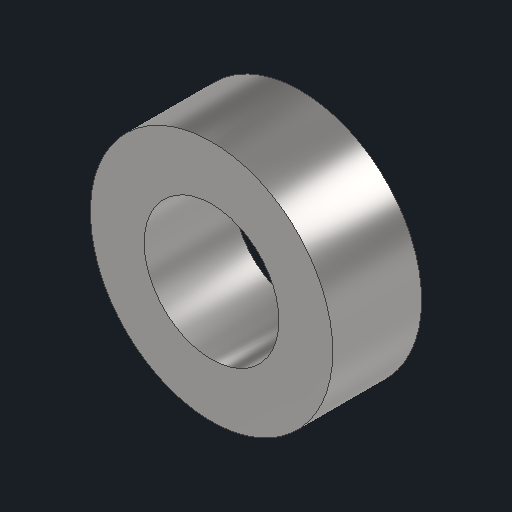
# Autodesk Inventor part: small_bearing
Saved by Autodesk Inventor 2023 (Build 270158000, 158)
## iProperties
Created: 2024-04-13
Part Number: small_bearing
Material: Steel, Alloy
Document SubType Name: Modeling
Designer: szymo
Density: 7.73 g/cm^3
Appearance: Semi-Polished
Mass: 1.12194 g
Surface Area: 2.33106 cm^2
Volume: 0.145142 cm^3
Author: szymo
Autodesk Inventor part; units mm, degrees
ref_plane "YZ Plane" through (0, 0, 0) normal (1, 0, 0) x (0, 1, 0)
ref_plane "XZ Plane" through (0, 0, 0) normal (0, 1, 0) x (-1, 0, 0)
ref_plane "XY Plane" through (0, 0, 0) normal (0, 0, 1) x (1, 0, 0)
sketch "Sketch1" plane through (0, 0, 0) normal (0, 0, 1) x (1, 0, 0)
  circle A0 centre (2.5, 0) radius 2.5 projected
  circle A1 centre (2.5, 0) radius 4.5
  point P0 (0, 0)
  dimension "d0" = 9
  constraints: 1 centre point, 1 coincident, 1 horizontal alignment
  measures "d0" diameter of A1
ref_plane "Work Plane1" through (-2.5, -5, -5) normal (0, 0, 1) x (1, 0, 0)
extrude "Extrusion2" add sketch "Sketch1" along normal blind 0.3 and the other way blind 3
body "Solid2"
